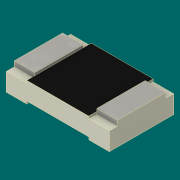
# Autodesk Inventor part: 0805
Saved by Autodesk Inventor 2016 (Build 200138000, 138)
## iProperties
Created: 2015-08-25
Part Number: 0805
Material: ABS Plastic
Document SubType Name: Modeling
Designer: Cosmic
Density: 1.06 g/cm^3
Appearance: Smooth - Ivory
Author: Cosmic
Autodesk Inventor part; units mm, degrees
ref_plane "YZ Plane" through (0, 0, 0) normal (1, 0, 0) x (0, 1, 0)
ref_plane "XZ Plane" through (0, 0, 0) normal (0, 1, 0) x (-1, 0, 0)
ref_plane "XY Plane" through (0, 0, 0) normal (0, 0, 1) x (1, 0, 0)
sketch "Sketch1" plane through (0, 0, 0) normal (0, 0, 1) x (1, 0, 0)
  line L0 (-1, -0.625) -> (1, -0.625)
  line L1 (1, -0.625) -> (1, 0.625)
  line L2 (1, 0.625) -> (-1, 0.625)
  line L3 (-1, 0.625) -> (-1, -0.625)
  line L4 (-1, -0.625) -> (1, 0.625) construction
  line L5 (1, -0.625) -> (-1, 0.625) construction
  point P0 (0, 0)
  dimension "d0" = 2
  dimension "d1" = 1.25
  constraints: 12 end point, 2 midpoint, 2 parallel, 1 horizontal, 1 perpendicular
  measures "d0" distance of L2.end L1.end
  measures "d1" distance of L1.end L0.end
extrude "Extrusion1" add sketch "Sketch1" along normal blind 0.45
sketch "Sketch2" plane through (0, 0, 0.45) normal (0, 0, 1) x (1, 0, 0)
  line L0 (-1, -0.625) -> (1, -0.625) projected
  line L1 (1, -0.625) -> (1, 0.625) projected
  line L2 (1, 0.625) -> (-1, 0.625) projected
  line L3 (-1, 0.625) -> (-1, -0.625) projected
  line L4 (-0.6, -0.625) -> (0.6, -0.625)
  line L5 (0.6, -0.625) -> (0.6, 0.625)
  line L6 (0.6, 0.625) -> (-0.6, 0.625)
  line L7 (-0.6, 0.625) -> (-0.6, -0.625)
  line L8 (-0.6, -0.625) -> (0.6, 0.625) construction
  line L9 (0.6, -0.625) -> (-0.6, 0.625) construction
  line L10 (0.6, -0.4688) -> (1, -0.4688)
  line L11 (1, -0.4688) -> (1, 0.4688)
  line L12 (1, 0.4688) -> (0.6, 0.4688)
  line L13 (0.6, 0.4688) -> (0.6, -0.4688)
  line L14 (-1, 0.625) -> (-1, -0.625) projected
  line L15 (-0.6, 0.4688) -> (-1, 0.4688)
  line L16 (-1, 0.4688) -> (-1, -0.4688)
  line L17 (-1, -0.4688) -> (-0.6, -0.4687)
  line L18 (-0.6, -0.4687) -> (-0.6, 0.4688)
  point P0 (0, 0)
  dimension "d4" = 0.4
  dimension "d5" = 0.9375
  dimension "d6" = 0.1562
  dimension "d7" = 0.9375
  dimension "d8" = 0.1562
  constraints: 28 end point, 6 parallel, 5 point on line, 3 horizontal, 3 perpendicular, 2 midpoint
  measures "d4" distance between parallel lines of L3 L7
  measures "d5" distance between parallel lines of L15 L17
  measures "d6" distance between parallel lines of L0 L17
  measures "d7" distance between parallel lines of L12 L10
  measures "d8" distance between parallel lines of L0 L10
extrude "Extrusion2" cut sketch "Sketch2" against normal blind 0.1 contours L3 L17 L7 L0 | L5 L10 L1 L0 | L3 L2 L7 L15 | L5 L2 L1 L12
sketch "Sketch3" plane through (0, 0, 0.45) normal (0, 0, 1) x (1, 0, 0)
  line L0 (-0.6, 0.625) -> (-0.6, 0.4688) projected
  line L1 (-0.6, 0.4688) -> (-1, 0.4688) projected
  line L2 (-1, 0.4688) -> (-1, -0.4688) projected
  line L3 (-1, -0.4688) -> (-0.6, -0.4687) projected
  line L4 (-0.6, -0.4687) -> (-0.6, -0.625) projected
  line L5 (-0.6, -0.625) -> (0.6, -0.625) projected
  line L6 (0.6, -0.625) -> (0.6, -0.4688) projected
  line L7 (0.6, -0.4688) -> (1, -0.4688) projected
  line L8 (1, -0.4688) -> (1, 0.4688) projected
  line L9 (1, 0.4688) -> (0.6, 0.4688) projected
  line L10 (0.6, 0.4688) -> (0.6, 0.625) projected
  line L11 (0.6, 0.625) -> (-0.6, 0.625) projected
  line L12 (0.6, 0.625) -> (-0.6, 0.625) projected
  line L13 (-0.6, -0.625) -> (0.6, -0.625)
  line L14 (0.6, -0.625) -> (0.6, 0.625)
  line L15 (0.6, 0.625) -> (-0.6, 0.625)
  line L16 (-0.6, 0.625) -> (-0.6, -0.625)
  line L17 (-0.6, -0.625) -> (0.6, 0.625) construction
  line L18 (0.6, -0.625) -> (-0.6, 0.625) construction
  point P0 (0, 0)
  constraints: 12 end point, 2 midpoint, 2 parallel, 1 horizontal, 1 perpendicular
extrude "Extrusion3" cut sketch "Sketch3" against normal blind 0.05 contours L11 L10 L14 L6 L5 L4 L16 L0
sketch "Sketch4" plane through (0, 0, 0) normal (0, 0, -1) x (-1, 0, 0)
  line L0 (1, -0.625) -> (-1, -0.625) projected
  line L1 (1, 0.625) -> (1, -0.625) projected
  line L2 (-1, 0.625) -> (1, 0.625) projected
  line L3 (-1, -0.625) -> (-1, 0.625) projected
  line L4 (-1, 0.625) -> (1, 0.625) projected
  line L5 (-1, 0.625) -> (-0.6, 0.625)
  line L6 (-0.6, 0.625) -> (-0.6, -0.625)
  line L7 (-0.6, -0.625) -> (-1, -0.625)
  line L8 (-1, -0.625) -> (-1, 0.625)
  line L9 (1, 0.625) -> (0.6, 0.625)
  line L10 (0.6, 0.625) -> (0.6, -0.625)
  line L11 (0.6, -0.625) -> (1, -0.625)
  line L12 (1, -0.625) -> (1, 0.625)
  point P0 (0, 0)
  dimension "d13" = 0.4
  dimension "d14" = 0.4
  constraints: 16 end point, 4 parallel, 2 horizontal, 2 perpendicular, 2 point on line
  measures "d13" distance between parallel lines of L1 L10
  measures "d14" distance between parallel lines of L3 L6
extrude "Extrusion4" cut sketch "Sketch4" against normal blind 0.05 contours L0 L6 L2 L10
equation "\"d7\" = d5"
equation "\"d8\" = d6"
body "Solid1"
